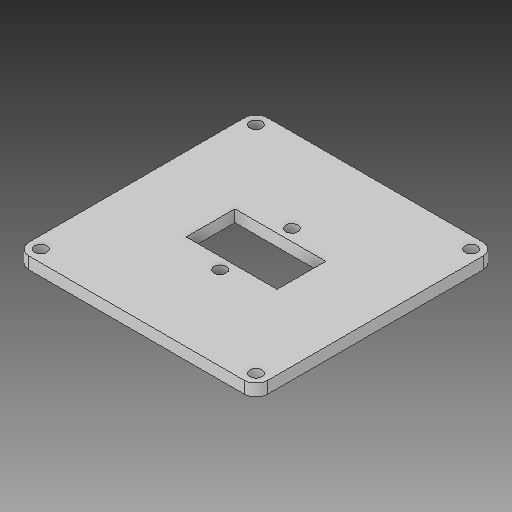
# Autodesk Inventor part: 板子5
Saved by Autodesk Inventor 2017 (Build 210142000, 142)
## iProperties
Part Number: 板子5
Material: 一般
Document SubType Name: Modeling
Designer: User
Density: 1 g/cm^3
Appearance: 預設
Author: User
Autodesk Inventor part; units mm, degrees
ref_plane "YZ Plane" through (0, 0, 0) normal (1, 0, 0) x (0, 1, 0)
ref_plane "XZ Plane" through (0, 0, 0) normal (0, 1, 0) x (-1, 0, 0)
ref_plane "XY Plane" through (0, 0, 0) normal (0, 0, 1) x (1, 0, 0)
sketch "草圖1" plane through (0, 0, 0) normal (0, 1, 0) x (-1, 0, 0)
  line L0 (30, 30) -> (-30, 30)
  line L1 (-30, 30) -> (-30, -30)
  line L2 (-30, -30) -> (30, -30)
  line L3 (30, -30) -> (30, 30)
  line L4 (30, 30) -> (30, 27)
  line L5 (30, 27) -> (27, 27)
  circle A0 centre (27, 27) radius 1.5
  circle A1 centre (-27, 27) radius 1.5
  circle A2 centre (-27, -27) radius 1.5
  circle A3 centre (27, -27) radius 1.5
  line L6 (11.4, 6.1) -> (-11.4, 6.1)
  line L7 (-11.4, 6.1) -> (-11.4, -6.1)
  line L8 (-11.4, -6.1) -> (11.4, -6.1)
  line L9 (11.4, -6.1) -> (11.4, 6.1)
  line L10 (0, 6.1) -> (0, 9)
  circle A4 centre (0, 9) radius 1.5
  line L11 (42, 0) -> (-42, 0) projected
  circle A5 centre (0, -9) radius 1.5
  line L12 (27, 27) -> (0, 0)
  dimension "d0" = 60
  dimension "d1" = 60
  dimension "d2" = 30
  dimension "d3" = 30
  dimension "d4" = 3
  dimension "d5" = 3
  dimension "d6" = 3
  dimension "d9" = 360
  dimension "d11" = 12.2
  dimension "d12" = 22.8
  dimension "d13" = 6.1
  dimension "d14" = 11.4
  dimension "d15" = 2.9
  dimension "d16" = 3
  constraints: 24 end point, 6 centre point, 4 parallel, 3 perpendicular, 2 coincident, 2 horizontal, 1 midpoint, 1 point on line, 1 symmetric about line, 1 vertical, 10 other
  measures "d0" distance of L1.end L2.end
  measures "d1" distance of L2.end L0.start
  measures "d2" distance from line of L12.end L2
  measures "d3" distance from line of L12.end L3
  measures "d4" distance of L0.start L4.end
  measures "d5" distance of L4.end L5.end
  measures "d6" diameter of A0
  measures "d11" distance of L8.end L6.start
  measures "d12" distance of L7.end L8.end
  measures "d13" distance from line of L12.end L8
  measures "d14" distance from line of L9 L12.end
  measures "d15" distance of L10.start L10.end
  measures "d16" diameter of A4
extrude "擠出1" add sketch "草圖1" along normal mid plane 3 contours L3 L5 A0 L12 L6 L7 L11 L1 L0 | L3 L11 L9 L6 L12 A0 L5 | L11 L7 L8 L9 L3 L2 L1
fillet "圓角1" radius 3 4 edges at (30, 0, 30) (-30, 0, 30) (-30, 0, -30) (30, 0, -30)
